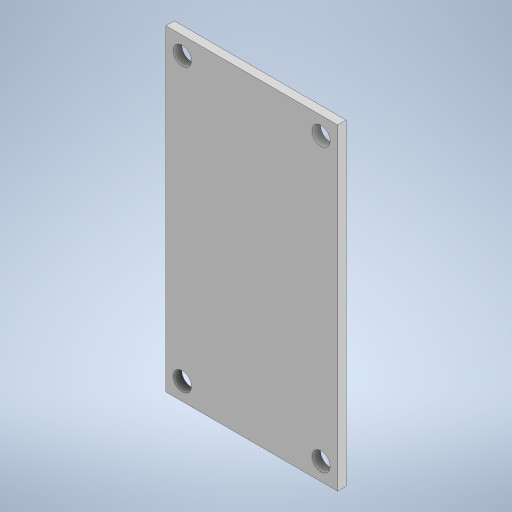
# Autodesk Inventor part: esp32f
Saved by Autodesk Inventor 2023 (Build 270158000, 158)
## iProperties
Created: 2022-06-24
Part Number: esp32f
Material: 일반
Document SubType Name: Modeling
Designer: user
Density: 1 g/cm^3
Appearance: 기본값
Author: user
Autodesk Inventor part; units mm, degrees
ref_plane "YZ Plane" through (0, 0, 0) normal (1, 0, 0) x (0, 1, 0)
ref_plane "XZ Plane" through (0, 0, 0) normal (0, 1, 0) x (-1, 0, 0)
ref_plane "XY Plane" through (0, 0, 0) normal (0, 0, 1) x (1, 0, 0)
sketch "스케치1" plane through (0, 0, 0) normal (0, 0, 1) x (1, 0, 0)
  line L0 (-15.6, 28.8) -> (15.6, 28.8)
  line L1 (15.6, 28.8) -> (15.6, -28.8)
  line L2 (15.6, -28.8) -> (-15.6, -28.8)
  line L3 (-15.6, -28.8) -> (-15.6, 28.8)
  line L4 (-15.6, 28.8) -> (15.6, -28.8) construction
  line L5 (15.6, 28.8) -> (-15.6, -28.8) construction
  circle A0 centre (-12.592, 25.5984) radius 1.653
  line L6 (0, 0) -> (0, 15.0785)
  line L7 (0, 0) -> (8.5646, 0)
  circle A1 centre (12.592, 25.5984) radius 1.653
  circle A2 centre (-12.592, -25.5984) radius 1.653
  circle A3 centre (12.592, -25.5984) radius 1.653
  dimension "d0" = 31.2
  dimension "d1" = 57.6
  constraints: 16 end point, 4 centre point, 3 symmetric about line, 2 horizontal, 2 midpoint, 2 parallel, 1 perpendicular, 1 vertical, 3 other
  measures "d0" distance of L1.end L2.end
  measures "d1" distance of L0.end L1.end
extrude "돌출1" add sketch "스케치1" along normal blind 1.53
